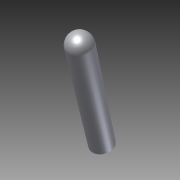
# Autodesk Inventor part: M2TSactu
Saved by Autodesk Inventor 2011 SP1 (Build 150282100, 282)
## iProperties
Created: 2013-12-24
Part Number: M2TSactu
Catalog Web Link: www.cadenas.de
Description: M2T Series - Process Sealed Miniature Toggles - Actuators-
Vendor: NKKSWITCHES
Document SubType Name: Modeling
Designer: PARTuser1
Manufacturer: NKKSWITCHES
Density: 1 g/cm^3
Category: PARTsolutions
Company: NKKSWITCHES
Title: M2TSactu
Author: Cadenas PARTsolutions
PSOL_IDENT_0: {$CADENAS_DATA\23d-libs\nkkswitches\toggle\m2t\parts\m2t_actuators.prj},213 {VTYP=3D},{NB=M2TSactu},
PSOL_IDENT_1: {LINA=M2TSactu},{NN=M2T Series - Process Sealed Miniature Toggles - Actuators},{DATE=07.04.2009 06:4
PSOL_IDENT_2: 9:49},{GEOMDATE=07.04.2009 06:40:00},{VERSION=},{LINEID=10},{LINESUBID=-1},{WBVAR=ACTU}  {NB=M2TSact
PSOL_IDENT_3: u},{LINA=M2TSactu},{KT=DUMMY},{PN=M2TS},{SRS=M2T},{ACTU=S}
CNS_NN: M2T Series - Process Sealed Miniature Toggles - Actuators
CNS_NB: M2TSactu
CNS_NBSYN: $PN.actu
CNS_LINA: M2TSactu
CNS_PN: M2TS
CNS_SRS: M2T
CNS_ACTU: S - .500" (12.7mm) Bat Lever
SUPPLIER: NKKSWITCHES
ARTICLENO: M2TSactu
BOMINFO: M2TSactu
CREATOR: CADENAS GmbH
Autodesk Inventor part; units mm, degrees
sketch "Sketch_1" plane through (0, 0, 0) normal (1, 0, 0) x (0, 1, 0)
  line L0 (-0.99, -0.2286) -> (12.3745, 2.8569)
  arc A0 (11.3079, 1.1772) -> (12.3745, 2.8569) centre (11.0133, 2.5428) ccw
  line L1 (11.3079, 1.1772) -> (-0.7157, -1.4165)
  line L2 (-0.7157, -1.4165) -> (-0.99, -0.2286)
  line L3 (-0.99, -0.2286) -> (12.3745, 2.8569)
  constraints: 8 end point, 2 point on circle, 1 centre point
revolve "Revolution1" add sketch "Sketch_1" angle 360 about axis through (0, -0.99, -0.2286) along (0, -0.9743701, -0.2249511)
ref_plane "bushing_XY" through (0, 0, 0) normal (0, 1, 0) x (1, 0, 0)
ref_plane "bushing_YZ" through (0, 0, 0) normal (1, 0, 0) x (0, 0, -1)
ref_plane "bushing_ZX" through (0, 0, 0) normal (0, 0, -1) x (0, 1, 0)
body "Solid1"
